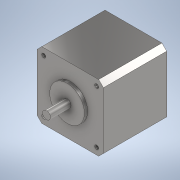
# Autodesk Inventor part: motor
Saved by Autodesk Inventor 2021.2 (Build 252289000, 289)
## iProperties
Created: 2024-04-19
Part Number: motor
Material: Iron, Malleable
Document SubType Name: Modeling
Designer: cioba
Density: 7.15 g/cm^3
Appearance: Semi-Polished
Author: cioba
Autodesk Inventor part; units mm, degrees
ref_plane "YZ Plane" through (0, 0, 0) normal (1, 0, 0) x (0, 1, 0)
ref_plane "XZ Plane" through (0, 0, 0) normal (0, 1, 0) x (-1, 0, 0)
ref_plane "XY Plane" through (0, 0, 0) normal (0, 0, 1) x (1, 0, 0)
sketch "Sketch1" plane through (0, 0, 0) normal (0, 0, 1) x (1, 0, 0)
  line L0 (-3.9016, 5.1111) -> (32.0984, 5.1111)
  line L1 (35.0984, 2.1111) -> (35.0984, -33.8889)
  line L2 (32.0984, -36.8889) -> (-3.9016, -36.8889)
  line L3 (-6.9016, -33.8889) -> (-6.9016, 2.1111)
  circle A0 centre (14.0984, -15.8889) radius 11
  circle A1 centre (14.0984, -15.8889) radius 2.5
  line L4 (35.0984, 2.1111) -> (32.0984, 5.1111)
  line L5 (-6.9016, 2.1111) -> (-3.9016, 5.1111)
  line L6 (-6.9016, -33.8889) -> (-3.9016, -36.8889)
  line L7 (35.0984, -33.8889) -> (32.0984, -36.8889)
  circle A2 centre (30.8484, -32.6389) radius 1.25
  circle A3 centre (-2.6516, -32.6389) radius 1.25
  circle A4 centre (-2.6516, 0.8611) radius 1.25
  circle A5 centre (30.8484, 0.8611) radius 1.25
  point P0 (0, 0)
  constraints: 16 end point, 6 centre point, 2 parallel, 1 coincident, 1 horizontal, 1 perpendicular
extrude "Extrusion1" add sketch "Sketch1" along normal blind 15 contours A1
extrude "Extrusion2" add sketch "Sketch1" along normal blind 2 contours A0
extrude "Extrusion3" add sketch "Sketch1" against normal blind 40 contours L0 L4 L1 L7 L2 L6 L3 L5 | A0 | A1 | A2 | A3 | A4 | A5
extrude "Extrusion4" cut sketch "Sketch1" against normal blind 5 contours A5
extrude "Extrusion5" cut sketch "Sketch1" against normal blind 5 contours A2
extrude "Extrusion6" cut sketch "Sketch1" against normal blind 5 contours A3
extrude "Extrusion7" cut sketch "Sketch1" against normal blind 5 contours A4
body "Solid1"
